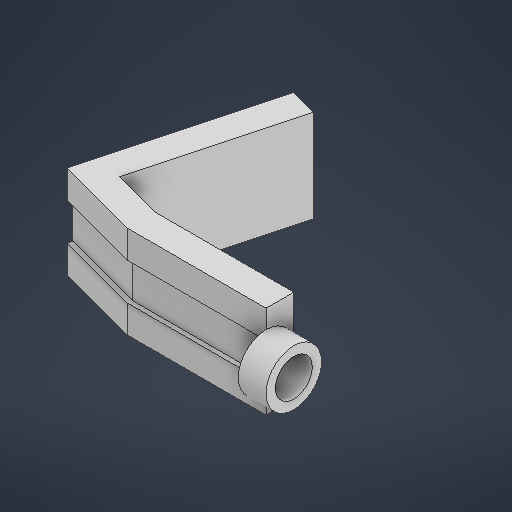
# Autodesk Inventor part: GY_906 Casetop
Saved by Autodesk Inventor 2027.1 (Build 311270010, 270A)
## iProperties
Created: 2026-09-10
Part Number: GY_906 Casetop
Material: Genérico
Document SubType Name: Modeling
Designer: marco
Density: 1 g/cm^3
Appearance: Valor por defecto
Author: marco
Autodesk Inventor part; units mm, degrees
ref_plane "YZ Plane" through (0, 0, 0) normal (1, 0, 0) x (0, 1, 0)
ref_plane "XZ Plane" through (0, 0, 0) normal (0, 1, 0) x (-1, 0, 0)
ref_plane "XY Plane" through (0, 0, 0) normal (0, 0, 1) x (1, 0, 0)
sketch "Boceto1" plane through (0, 0, 0) normal (0, 1, 0) x (-1, 0, 0)
  line L0 (0, 0) -> (-15, 0)
  line L1 (0, 0) -> (7.0223, -1.8816)
  line L2 (0, 0) -> (7.27, 0) construction
  line L3 (8.8653, -2.3754) -> (7.0223, -1.8816)
  line L4 (8.8653, -2.3754) -> (3.6889, -21.694)
  line L5 (8.8653, -2.3754) -> (28.8653, -2.3754) construction
  line L6 (-15, 0) -> (-15, -3)
  line L7 (-15, -3) -> (0, -3)
  line L8 (0, -3) -> (5.2175, -4.398)
  line L9 (5.2175, -4.398) -> (25.2175, -4.398) construction
  line L10 (3.6889, -21.694) -> (0.7911, -20.9175)
  line L11 (0.7911, -20.9175) -> (5.2175, -4.398)
  point P0 (4.2275, -19.6837)
  dimension "d0" = 15
  dimension "d1" = 7.27
  dimension "d2" = 15
  dimension "d3" = 1.908
  dimension "d4" = 20
  dimension "d5" = 105
  dimension "d7" = 3
  constraints: 24 end point, 4 horizontal, 2 equal length, 2 perpendicular, 1 collinear, 1 point on line, 1 vertical
  measures "d0" distance of L0.start L0.end
  measures "d1" distance of L0.start L1.end
  measures "d2" angle of L1 L2
  measures "d3" distance of L1.end L3.start
  measures "d4" distance of L3.start L4.end
  measures "d5" angle of L4 L5
  measures "d7" distance of L0.end L6.end
extrude "Extrusión1" add sketch "Boceto1" along normal blind 10
sketch "Boceto2" plane through (0, 0, 0) normal (-0.258819, 0, 0.9659258) x (0.9659258, 0, 0.258819)
  line L0 (-9.178, 0) -> (-9.178, 10) projected
  line L1 (-9.178, 0) -> (-9.178, 3)
  line L2 (-9.178, 3) -> (0, 3)
  line L3 (0, 3) -> (0, 7)
  line L4 (0, 7) -> (-9.178, 7)
  line L5 (-9.178, 7) -> (-9.178, 3)
  point P0 (0, 0)
  dimension "d12" = 3
  dimension "d13" = 4
  constraints: 10 end point, 4 perpendicular, 2 point on line
  measures "d12" distance of L0.start L1.end
  measures "d13" distance of L2.end L3.end
extrude "Extrusión2" cut sketch "Boceto2" against normal blind 0.5
sketch "Boceto3" plane through (0, 0, 0) normal (0, 0, 1) x (1, 0, 0)
  line L0 (0, 0) -> (0, 3) projected
  line L1 (0, 3) -> (15, 3)
  line L2 (15, 0) -> (15, 10) projected
  line L3 (0, 7) -> (0, 10) projected
  line L4 (0, 7) -> (15, 7)
  line L5 (15, 7) -> (15, 3.2945)
  line L6 (15, 3.2945) -> (15, 3)
  line L7 (0, 7) -> (0, 3)
  line L8 (0, 0) -> (0, 10) projected
  point P0 (0.1294, 7)
  point P1 (0.1294, 3)
  constraints: 10 end point, 2 horizontal, 2 perpendicular, 1 collinear, 1 point on line
extrude "Extrusión3" cut sketch "Boceto3" against normal blind 0.5
sketch "Boceto4" plane through (15, 0, 0) normal (1, 0, 0) x (0, 0, -1)
  circle A0 centre (0, 5) radius 3
  circle A1 centre (0, 5) radius 2.5
  point P0 (0, 0)
  dimension "d18" = 6
  dimension "d19" = 5
  constraints: 2 centre point, 1 coincident
  measures "d18" diameter of A0
  measures "d19" diameter of A1
extrude "Extrusión4" add sketch "Boceto4" along normal blind 3 contours A0 | A1
sketch "Boceto5" plane through (18, 5, 0) normal (1, 0, 0) x (0, 0, -1)
  line L0 (0, 2) -> (0, 3) projected
  circle A0 centre (0, 0) radius 2
  point P0 (0, -5)
  dimension "d22" = 4
  constraints: 1 vertical alignment, 2 other
extrude "Extrusión5" cut sketch "Boceto5" against normal blind 3
